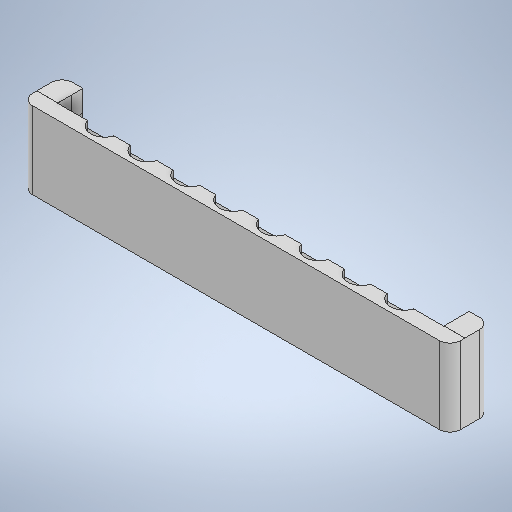
# Autodesk Inventor part: plate holder
Saved by Autodesk Inventor 2025.1 (Build 291241020, 241B)
## iProperties
Created: 2024-12-05
Part Number: plate holder
Material: Generic
Document SubType Name: Modeling
Designer: Hunter Mathis
Density: 1 g/cm^3
Appearance: Default
Author: Hunter Mathis
Autodesk Inventor part; units mm, degrees
ref_plane "YZ Plane" through (0, 0, 0) normal (1, 0, 0) x (0, 1, 0)
ref_plane "XZ Plane" through (0, 0, 0) normal (0, 1, 0) x (-1, 0, 0)
ref_plane "XY Plane" through (0, 0, 0) normal (0, 0, 1) x (1, 0, 0)
sketch "Sketch1" plane through (0, 0, 0) normal (0, 1, 0) x (-1, 0, 0)
  line L0 (63.5, -2.2225) -> (-63.5, -2.2225)
  line L1 (-63.5, -2.2225) -> (-63.5, 2.2225)
  line L2 (-63.5, 2.2225) -> (63.5, 2.2225)
  line L3 (63.5, 2.2225) -> (63.5, -2.2225)
  line L4 (63.5, -2.2225) -> (-63.5, 2.2225) construction
  line L5 (-63.5, -2.2225) -> (63.5, 2.2225) construction
  point P0 (0, 0)
  dimension "d0" = 127
  dimension "d1" = 4.445
  constraints: 12 end point, 2 midpoint, 2 parallel, 1 horizontal, 1 perpendicular
  measures "d0" distance of L1.end L2.end
  measures "d1" distance of L0.end L1.end
extrude "Extrusion1" add sketch "Sketch1" along normal blind 31.75
sketch "Sketch2" plane through (63.5, 0, -2.2225) normal (0, 0, -1) x (-1, 0, 0)
  line L0 (127, 0) -> (0, 0) projected
  line L1 (0, 0) -> (127, 0)
  line L2 (127, 0) -> (127, 25.4116)
  line L3 (127, 25.4116) -> (0, 25.4116)
  line L4 (0, 25.4116) -> (0, 0)
  point P0 (63.5, 0)
  constraints: 8 end point, 3 equal length, 1 perpendicular
extrude "Extrusion2" add sketch "Sketch2" along normal blind 7.4676
sketch "Sketch3" plane through (-63.5, 25.4116, -2.2225) normal (0, 1, 0) x (1, 0, 0)
  point P0 (63.5, -2.2225)
sketch "Sketch4" plane through (63.5, 0, -9.6901) normal (0, 0, -1) x (-1, 0, 0)
  line L0 (0, 25.4116) -> (0, 0) projected
  line L1 (6.223, 12.7058) -> (6.223, 25.4116)
  line L2 (0, 25.4116) -> (6.223, 25.4116)
  line L3 (0, 25.4116) -> (0, 12.7058)
  line L4 (0, 12.7058) -> (0, 3.1808)
  line L5 (0, 0) -> (0, 31.75) projected
  line L6 (0, 3.1808) -> (6.223, 3.1808)
  line L7 (6.223, 3.1808) -> (6.223, 12.7058)
  line L8 (0, 25.4116) -> (127, 25.4116) projected
  line L9 (127, 0) -> (127, 25.4116) projected
  line L10 (120.777, 12.7058) -> (120.777, 25.4116)
  line L11 (6.223, 25.4116) -> (120.777, 25.4116)
  line L12 (120.777, 12.7058) -> (120.777, 3.1808)
  line L13 (120.777, 3.1808) -> (127, 3.1808)
  line L14 (127, 3.1808) -> (127, 25.4116)
  line L15 (127, 0) -> (127, 31.75) projected
  line L16 (6.223, 3.1808) -> (120.777, 3.1808)
  line L17 (6.223, 3.1808) -> (6.223, 22.2308)
  line L18 (120.777, 22.2308) -> (6.223, 22.2308)
  line L19 (120.777, 22.2308) -> (120.777, 3.1808)
  line L20 (6.223, 3.1808) -> (120.777, 3.1808)
  point P0 (63.5, 0)
  point P1 (6.223, 22.2308)
  dimension "d6" = 6.223
  dimension "d7" = 9.525
  dimension "d13" = 6.223
  dimension "d14" = 19.05
  constraints: 32 end point, 5 collinear, 5 point on line, 4 perpendicular, 1 horizontal, 1 midpoint, 1 parallel, 1 vertical
  measures "d6" distance of L3.end L1.start
  measures "d7" distance of L3.end L4.end
  measures "d13" distance of L12.end L13.end
  measures "d14" distance between parallel lines of L18 L16
extrude "Extrusion3" cut sketch "Sketch4" against normal blind 4.699 contours L8 L10 L18 L1 | L18 L10 L12 L16 L7 L1
extrude "Extrusion4" add sketch "Sketch4" against normal blind 1.143 contours L18 L10 L12 L16 L7 L1
sketch "Sketch5" plane through (-63.5, 25.4116, -2.2225) normal (0, 1, 0) x (1, 0, 0)
  point P0 (63.5, -2.2225)
sketch "Sketch6" plane through (-63.5, 25.4116, -2.2225) normal (0, 1, 0) x (1, 0, 0)
  point P0 (63.5, -2.2225)
sketch "Sketch7" plane through (63.5, 0, 2.2225) normal (1, 0, 0) x (0, 0, -1)
  line L0 (0, 0) -> (0, 12.7)
  line L1 (0, 0) -> (0, 31.75) projected
  line L2 (0, 12.7) -> (11.9126, 12.7)
  line L3 (10.7696, 22.2308) -> (10.7696, 3.1808) projected
  line L4 (11.9126, 25.4116) -> (11.9126, 0) projected
  line L5 (11.9126, 12.7) -> (11.9126, 0)
  line L6 (0, 0) -> (11.9126, 0) projected
  line L7 (11.9126, 0) -> (0, 0)
  point P0 (2.2225, 0)
  dimension "d26" = 12.7
  constraints: 8 end point, 2 perpendicular, 1 collinear, 1 point on line
  measures "d26" distance of L0.start L0.end
extrude "Extrusion6" cut sketch "Sketch7" against normal through all
sketch "Sketch8" plane through (63.5, 12.7, -9.6901) normal (0, -1, 0) x (1, 0, 0)
  line L0 (-127, 11.9126) -> (0, 11.9126) projected
  line L1 (0, 7.4676) -> (0, 0) projected
  line L2 (0, 11.9126) -> (0, 0)
  line L3 (0, 0) -> (-127, 0)
  line L4 (-127, 0) -> (-127, 11.9126)
  line L5 (-127, 11.9126) -> (0, 11.9126)
  point P0 (-63.5, 9.6901)
  point P1 (-127, 11.9126)
  constraints: 8 end point, 2 parallel, 1 collinear, 1 perpendicular
extrude "Extrusion7" add sketch "Sketch8" along normal blind 3.81
sketch "Sketch9" plane through (-63.5, 25.4116, -2.2225) normal (0, 1, 0) x (1, 0, 0)
  line L0 (120.777, 2.7686) -> (6.223, 2.7686) projected
  line L1 (127, 0) -> (0, 0) projected
  line L2 (120.777, 2.7686) -> (6.5121, 2.7686)
  line L3 (6.5121, 0) -> (120.777, 0)
  line L4 (120.777, 2.7686) -> (120.777, 0)
  line L5 (120.777, 0) -> (6.223, 0)
  line L6 (6.223, 0) -> (6.223, 2.7686)
  line L7 (6.223, 2.7686) -> (120.777, 2.7686)
  line L8 (120.777, 6.3246) -> (120.777, 2.7686) projected
  point P0 (63.5, -2.2225)
  point P1 (6.223, 2.7686)
  constraints: 12 end point, 2 parallel, 1 collinear, 1 horizontal, 1 perpendicular, 1 point on line
extrude "Extrusion8" cut sketch "Sketch9" against normal blind 12.7
sketch "Sketch10" plane through (63.5, 12.7, -9.6901) normal (0, 1, 0) x (1, 0, 0)
  line L0 (-6.223, 0) -> (-6.223, -1.143) projected
  line L1 (-6.223, -1.143) -> (-6.223, -4.699) projected
  line L2 (-6.223, -1.143) -> (-6.223, -2.286)
  line L3 (-120.523, -2.286) -> (-120.523, -1.143)
  point P0 (-63.5, -9.6901)
  point P1 (-6.223, -7.4676)
  constraints: 4 end point, 1 parallel, 1 point on line
sketch "Sketch16" plane through (63.5, 0, -8.5471) normal (0, 0, 1) x (1, 0, 0)
  line L0 (-6.223, 22.2308) -> (-6.223, 12.7) projected
  line L1 (-6.223, 12.7) -> (-6.223, 22.2308)
  line L2 (-6.223, 22.2308) -> (-120.777, 22.2308)
  line L3 (-120.777, 22.2308) -> (-120.777, 12.7)
  line L4 (-120.777, 12.7) -> (-6.223, 12.7)
  point P0 (-63.5, 0)
  constraints: 8 end point, 2 parallel, 1 perpendicular, 1 vertical
extrude "Extrusion14" add sketch "Sketch16" along normal blind 2.4892
sketch "Sketch11" plane through (63.5, 8.89, -9.6901) normal (0, -1, 0) x (1, 0, 0)
  line L0 (0, 11.9126) -> (0, 7.4676) projected
  line L1 (0, 11.9126) -> (0, 7.4676)
  line L2 (0, 7.4676) -> (-6.35, 7.4676)
  line L3 (0, 11.9126) -> (-127, 11.9126) projected
  line L4 (-6.35, 11.9126) -> (-6.35, 5.5626)
  circle A0 centre (-6.35, 5.5626) radius 2.3241
  circle A1 centre (-19.05, 5.5626) radius 2.3241
  circle A2 centre (-31.75, 5.5626) radius 2.3241
  circle A3 centre (-44.45, 5.5626) radius 2.3241
  circle A4 centre (-57.15, 5.5626) radius 2.3241
  circle A5 centre (-69.85, 5.5626) radius 2.3241
  circle A6 centre (-82.55, 5.5626) radius 2.3241
  circle A7 centre (-95.25, 5.5626) radius 2.3241
  circle A8 centre (-107.95, 5.5626) radius 2.3241
  circle A9 centre (-120.65, 5.5626) radius 2.3241
  circle A10 centre (-6.35, 5.5626) radius 4.1275
  circle A11 centre (-19.05, 5.5626) radius 4.1275
  circle A12 centre (-31.75, 5.5626) radius 4.1275
  circle A13 centre (-44.45, 5.5626) radius 4.1275
  circle A14 centre (-57.15, 5.5626) radius 4.1275
  circle A15 centre (-69.85, 5.5626) radius 4.1275
  circle A16 centre (-82.55, 5.5626) radius 4.1275
  circle A17 centre (-95.25, 5.5626) radius 4.1275
  line L5 (-127, 11.9126) -> (-127, 0) projected
  line L6 (-127, 0) -> (-127, 11.9126)
  line L7 (-127, 5.9563) -> (0, 5.9563)
  circle A18 centre (-6.35, 6.35) radius 2.3241
  circle A19 centre (-19.05, 6.35) radius 2.3241
  circle A20 centre (-31.75, 6.35) radius 2.3241
  circle A21 centre (-44.45, 6.35) radius 2.3241
  circle A22 centre (-57.15, 6.35) radius 2.3241
  circle A23 centre (-69.85, 6.35) radius 2.3241
  circle A24 centre (-82.55, 6.35) radius 2.3241
  circle A25 centre (-95.25, 6.35) radius 2.3241
  circle A26 centre (-107.95, 6.35) radius 2.3241
  circle A27 centre (-120.65, 6.35) radius 2.3241
  point P0 (-63.5, 9.6901)
  dimension "d38" = 6.35
  dimension "d39" = 4.6482
  dimension "d42" = 12.7
  dimension "d51" = 8.255
  dimension "d54" = 12.7
  constraints: 28 centre point, 10 end point, 10 symmetric about line, 3 horizontal, 2 coincident, 2 perpendicular, 1 collinear, 1 midpoint, 1 point on line, 1 vertical, 42 other
  measures "d38" distance of L4.start L4.end
  measures "d39" diameter of A0
  measures "d42" distance of A0.centre A1.centre
  measures "d51" diameter of A10
  measures "d54" distance of A10.centre A11.centre
sketch "Sketch13" plane through (63.5, 12.7, -9.6901) normal (0, 1, 0) x (1, 0, 0)
  circle A0 centre (-19.05, -5.5626) radius 2.3241 projected
  circle A1 centre (-19.05, -5.5626) radius 4.1275
  line L0 (-6.223, -1.143) -> (-120.777, -1.143) projected
  line L1 (-6.223, -3.6322) -> (-6.223, -4.699) projected
  line L2 (-120.777, -4.699) -> (-120.777, -3.6322) projected
  circle A2 centre (-31.75, -5.5626) radius 4.1275
  circle A3 centre (-44.45, -5.5626) radius 4.1275
  circle A4 centre (-57.15, -5.5626) radius 4.1275
  circle A5 centre (-69.85, -5.5626) radius 4.1275
  circle A6 centre (-82.55, -5.5626) radius 4.1275
  circle A7 centre (-95.25, -5.5626) radius 4.1275
  circle A8 centre (-107.95, -5.5626) radius 4.1275
  line L3 (-6.223, -4.699) -> (-120.777, -4.699) projected
  line L4 (-6.223, -3.6322) -> (-120.777, -3.6322) projected
  line L5 (-127, -11.9126) -> (0, -11.9126) projected
  line L6 (0, 0) -> (0, -11.9126)
  line L7 (0, -11.9126) -> (0, -5.9563)
  line L8 (-127, -11.9126) -> (-127, 0) projected
  line L9 (0, -5.9563) -> (-2.9666, -5.9563)
  circle A9 centre (-19.05, -6.35) radius 2.3241
  circle A10 centre (-19.05, -6.35) radius 4.1275
  line L10 (-6.223, -10.7696) -> (-120.777, -10.7696)
  line L11 (-6.223, -8.2804) -> (-6.223, -7.2136)
  line L12 (-120.777, -7.2136) -> (-120.777, -8.2804)
  circle A11 centre (-31.75, -6.35) radius 4.1275
  circle A12 centre (-44.45, -6.35) radius 4.1275
  circle A13 centre (-57.15, -6.35) radius 4.1275
  circle A14 centre (-69.85, -6.35) radius 4.1275
  circle A15 centre (-82.55, -6.35) radius 4.1275
  circle A16 centre (-95.25, -6.35) radius 4.1275
  circle A17 centre (-107.95, -6.35) radius 4.1275
  line L13 (-6.223, -7.2136) -> (-120.777, -7.2136)
  line L14 (-6.223, -8.2804) -> (-120.777, -8.2804)
  line L15 (-127, 0) -> (-127, -11.9126)
  point P0 (-63.5, -9.6901)
  point P1 (-63.5, -2.2225)
  dimension "d59" = 8.255
  dimension "d62" = 12.7
  constraints: 18 end point, 18 symmetric about line, 17 centre point, 2 coincident, 1 horizontal, 1 midpoint, 1 vertical, 9 other
  measures "d59" diameter of A1
  measures "d62" distance of A1.centre A2.centre
fillet "Fillet1" radius 3.175 4 edges at (63.5, 20.32, 2.2225) (63.5, 17.1508, -9.6901) (-63.5, 17.1508, -9.6901) (-63.5, 20.32, 2.2225)
sketch "Sketch17" plane through (57.277, 25.4116, -2.2225) normal (0, 1, 0) x (1, 0, 0)
  line L0 (6.223, 0) -> (0, 0) projected
  line L1 (6.223, 4.2926) -> (6.223, -1.27) projected
  line L2 (6.223, 0) -> (6.223, 4.2926)
  arc A0 (6.223, 4.2926) -> (3.048, 7.4676) centre (3.048, 4.2926) ccw projected
  arc A1 (6.223, 4.2926) -> (3.048, 7.4676) centre (3.048, 4.2926) ccw
  line L3 (3.048, 7.4676) -> (0, 7.4676)
  line L4 (0, 7.4676) -> (0, 0) projected
  line L5 (0, 0) -> (6.223, 0)
  point P0 (-57.277, -2.2225)
  constraints: 6 end point, 2 point on circle, 1 centre point, 1 collinear, 1 tangent, 1 vertical
extrude "Extrusion15" add sketch "Sketch17" along normal blind 6.35
sketch "Sketch18" plane through (-63.5, 25.4116, -2.2225) normal (0, 1, 0) x (1, 0, 0)
  line L0 (127, 0) -> (0, 0) projected
  line L1 (6.2253, 0) -> (6.2253, 7.4056)
  line L2 (3.175, 7.4676) -> (6.223, 7.4676) projected
  line L3 (6.223, 7.4676) -> (3.175, 7.4676)
  arc A0 (3.175, 7.4676) -> (0, 4.2926) centre (3.175, 4.2926) ccw projected
  line L4 (0, 4.2926) -> (0, 0)
  line L5 (0, -1.27) -> (0, 4.2926) projected
  line L6 (0, 0) -> (6.2253, 0)
  arc A1 (3.175, 7.4676) -> (0, 4.2926) centre (3.175, 4.2926) ccw
  line L7 (6.223, 7.4676) -> (6.2253, 3.7028)
  line L8 (6.2253, 0) -> (0, 0)
  line L9 (0, 4.2926) -> (0, 0)
  point P0 (63.5, -2.2225)
  point P1 (15.3884, 0)
  constraints: 14 end point, 4 collinear, 3 point on circle, 1 centre point, 1 concentric, 1 horizontal, 1 midpoint, 1 point on line, 1 vertical
extrude "Extrusion16" add sketch "Sketch18" along normal blind 6.35
extrude "Extrusion17" cut sketch "Sketch11" along normal through all both and the other way through all contours L7 A1 | A19 L7 | A1 A19 | A26 A8 | A8 L7 | L7 A26 | L7 A2 | A20 L7 | A2 A20 | A25 A7 | A7 L7 | L7 A25 | L7 A3 | A21 L7 | A3 A21 | A24 A6 | A6 L7 | L7 A24 | L7 A4 | A22 L7 | A4 A22 | A23 A5 | A5 L7 | L7 A23 picked at (-19.2951, 8.1254) picked at (-108.1951, 8.1254) picked at (-31.9951, 8.1254) picked at (-95.4951, 8.1254) picked at (-44.6951, 8.1254) picked at (-82.7951, 8.1254) picked at (-57.3951, 8.1254) picked at (-70.0951, 8.1254)
ref_plane "Work Plane1" through (44.45, 22.2308, -4.1275) normal (0, 1, 0) x (1, 0, 0)
sketch "Sketch19" plane through (44.45, 22.2308, -4.1275) normal (0, 1, 0) x (1, 0, 0)
  line L0 (12.827, 1.9304) -> (-101.727, 1.9304) projected
  arc A0 (-1.6357, 0.8636) -> (-2.0377, -1.905) centre (0, -0.7874) ccw projected
  line L1 (-23.7643, 0.8636) -> (-14.3357, 0.8636) projected
  arc A1 (-1.6357, 0.8636) -> (-2.0377, -1.905) centre (0, -0.7874) ccw projected
  line L2 (-23.7643, 0.8636) -> (-14.3357, 0.8636) projected
  line L3 (-101.727, 5.5626) -> (12.827, 5.5626) projected
  line L4 (-101.727, 1.9304) -> (-101.727, 5.5626) projected
  line L5 (12.827, 5.5626) -> (12.827, 1.9304) projected
  arc A2 (-23.3623, -1.905) -> (-23.7643, 0.8636) centre (-25.4, -0.7874) ccw projected
  line L6 (-14.7377, -1.905) -> (-23.3623, -1.905) projected
  arc A3 (-14.3357, 0.8636) -> (-14.7377, -1.905) centre (-12.7, -0.7874) ccw projected
  arc A4 (-74.1623, -1.905) -> (-74.5643, 0.8636) centre (-76.2, -0.7874) ccw projected
  line L7 (-65.5377, -1.905) -> (-74.1623, -1.905) projected
  arc A5 (-65.1357, 0.8636) -> (-65.5377, -1.905) centre (-63.5, -0.7874) ccw projected
  line L8 (-74.5643, 0.8636) -> (-65.1357, 0.8636) projected
  arc A6 (-61.4623, -1.905) -> (-61.8643, 0.8636) centre (-63.5, -0.7874) ccw projected
  line L9 (-52.8377, -1.905) -> (-61.4623, -1.905) projected
  arc A7 (-52.4357, 0.8636) -> (-52.8377, -1.905) centre (-50.8, -0.7874) ccw projected
  line L10 (-61.8643, 0.8636) -> (-52.4357, 0.8636) projected
  arc A8 (-10.6623, -1.905) -> (-11.0643, 0.8636) centre (-12.7, -0.7874) ccw projected
  line L11 (-2.0377, -1.905) -> (-10.6623, -1.905) projected
  line L12 (-11.0643, 0.8636) -> (-1.6357, 0.8636) projected
  arc A9 (-27.0357, 0.8636) -> (-27.4377, -1.905) centre (-25.4, -0.7874) ccw projected
  line L13 (-36.4643, 0.8636) -> (-27.0357, 0.8636) projected
  arc A10 (-36.0623, -1.905) -> (-36.4643, 0.8636) centre (-38.1, -0.7874) ccw projected
  line L14 (-27.4377, -1.905) -> (-36.0623, -1.905) projected
  arc A11 (-77.8357, 0.8636) -> (-78.2377, -1.905) centre (-76.2, -0.7874) ccw projected
  line L15 (-87.2643, 0.8636) -> (-77.8357, 0.8636) projected
  arc A12 (-86.8623, -1.905) -> (-87.2643, 0.8636) centre (-88.9, -0.7874) ccw projected
  line L16 (-78.2377, -1.905) -> (-86.8623, -1.905) projected
  arc A13 (-39.7357, 0.8636) -> (-40.1377, -1.905) centre (-38.1, -0.7874) ccw projected
  line L17 (-49.1643, 0.8636) -> (-39.7357, 0.8636) projected
  arc A14 (-48.7623, -1.905) -> (-49.1643, 0.8636) centre (-50.8, -0.7874) ccw projected
  line L18 (-40.1377, -1.905) -> (-48.7623, -1.905) projected
  arc A15 (2.0377, -1.905) -> (1.6357, 0.8636) centre (0, -0.7874) ccw projected
  line L19 (12.827, -1.905) -> (2.0377, -1.905) projected
  line L20 (12.827, 0.8636) -> (12.827, -1.905) projected
  line L21 (1.6357, 0.8636) -> (12.827, 0.8636) projected
  arc A16 (-90.5357, 0.8636) -> (-90.9377, -1.905) centre (-88.9, -0.7874) ccw projected
  line L22 (-101.727, 0.8636) -> (-90.5357, 0.8636) projected
  line L23 (-101.727, -1.905) -> (-101.727, 0.8636) projected
  line L24 (-90.9377, -1.905) -> (-101.727, -1.905) projected
  arc A17 (-23.3623, -1.905) -> (-23.7643, 0.8636) centre (-25.4, -0.7874) ccw projected
  line L25 (-14.7377, -1.905) -> (-23.3623, -1.905) projected
  arc A18 (-14.3357, 0.8636) -> (-14.7377, -1.905) centre (-12.7, -0.7874) ccw projected
  arc A19 (-74.1623, -1.905) -> (-74.5643, 0.8636) centre (-76.2, -0.7874) ccw projected
  line L26 (-65.5377, -1.905) -> (-74.1623, -1.905) projected
  arc A20 (-65.1357, 0.8636) -> (-65.5377, -1.905) centre (-63.5, -0.7874) ccw projected
  line L27 (-74.5643, 0.8636) -> (-65.1357, 0.8636) projected
  arc A21 (-61.4623, -1.905) -> (-61.8643, 0.8636) centre (-63.5, -0.7874) ccw projected
  line L28 (-52.8377, -1.905) -> (-61.4623, -1.905) projected
  arc A22 (-52.4357, 0.8636) -> (-52.8377, -1.905) centre (-50.8, -0.7874) ccw projected
  line L29 (-61.8643, 0.8636) -> (-52.4357, 0.8636) projected
  arc A23 (-10.6623, -1.905) -> (-11.0643, 0.8636) centre (-12.7, -0.7874) ccw projected
  line L30 (-2.0377, -1.905) -> (-10.6623, -1.905) projected
  line L31 (-11.0643, 0.8636) -> (-1.6357, 0.8636) projected
  arc A24 (-27.0357, 0.8636) -> (-27.4377, -1.905) centre (-25.4, -0.7874) ccw projected
  line L32 (-36.4643, 0.8636) -> (-27.0357, 0.8636) projected
  arc A25 (-36.0623, -1.905) -> (-36.4643, 0.8636) centre (-38.1, -0.7874) ccw projected
  line L33 (-27.4377, -1.905) -> (-36.0623, -1.905) projected
  arc A26 (-77.8357, 0.8636) -> (-78.2377, -1.905) centre (-76.2, -0.7874) ccw projected
  line L34 (-87.2643, 0.8636) -> (-77.8357, 0.8636) projected
  arc A27 (-86.8623, -1.905) -> (-87.2643, 0.8636) centre (-88.9, -0.7874) ccw projected
  line L35 (-78.2377, -1.905) -> (-86.8623, -1.905) projected
  arc A28 (-39.7357, 0.8636) -> (-40.1377, -1.905) centre (-38.1, -0.7874) ccw projected
  line L36 (-49.1643, 0.8636) -> (-39.7357, 0.8636) projected
  arc A29 (-48.7623, -1.905) -> (-49.1643, 0.8636) centre (-50.8, -0.7874) ccw projected
  line L37 (-40.1377, -1.905) -> (-48.7623, -1.905) projected
  arc A30 (2.0377, -1.905) -> (1.6357, 0.8636) centre (0, -0.7874) ccw projected
  line L38 (12.827, -1.905) -> (2.0377, -1.905) projected
  line L39 (12.827, 0.8636) -> (12.827, -1.905) projected
  line L40 (1.6357, 0.8636) -> (12.827, 0.8636) projected
  arc A31 (-90.5357, 0.8636) -> (-90.9377, -1.905) centre (-88.9, -0.7874) ccw projected
  line L41 (-101.727, 0.8636) -> (-90.5357, 0.8636) projected
  line L42 (-101.727, -1.905) -> (-101.727, 0.8636) projected
  line L43 (-90.9377, -1.905) -> (-101.727, -1.905) projected
  point P0 (-44.45, -4.1275)
extrude "Extrusion19" cut sketch "Sketch13" along normal blind 19.05 and the other way blind 2.54 contours A0 A9 L3 | A0 L3 A10 A1 L13 A9 | L3 A9 A0 L4 | A0 L4 A10 L3 | A9 L13 A0 | A0 L13 A9 L3 | L4 A0 | A0 L4 A10 | L3 A9 | L13 A9 L14 A0 | A0 L13 | A0 L3 A10 L4 | A10 L13 A1 | A9 A0 L3 | L13 A9 A0 | L13 A1 L14 A9 | A0 A9 L13 A1 A10 L3 | L13 A10 L14 A1 | A9 L14 A1 L13 | L14 A1 A9 | A9 L14 | L14 A10 A1 | L13 A10 A1 | A1 L14 A10 L13 | A11 L3 L4 | L4 A11 | L13 A2 A11 | A11 L14 A2 L13 | A11 A2 L13 L3 | A11 L14 A2 | A2 L14 L13 | A2 L13 A11 | A12 L3 L4 | L4 A12 | A11 L13 A2 L14 | A2 L14 | A12 A3 L13 L3 | L14 A3 L13 A12 | A12 L14 A3 | L13 A3 A12 | A3 L13 A12 | A13 L3 L4 | L4 A13 | A12 L13 A3 L14 | L14 A3 L13 | A3 L14 | A13 A4 L13 L3 | L14 A4 L13 A13 | A13 L14 A4 | L13 A4 A13 | A4 L13 A13 | A14 L3 L4 | L4 A14 | A13 L13 A4 L14 | L14 A4 L13 | A4 L14 | A14 A5 L13 L3 | L14 A5 L13 A14 | A14 L14 A5 | L13 A5 A14 | A5 L13 A14 | A15 L3 L4 | L4 A15 | A14 L13 A5 L14 | L14 A5 L13 | A5 L14 | A15 A6 L13 L3 | L14 A6 L13 A15 | A15 L14 A6 | L13 A6 A15 | A6 L13 A15 | A16 L3 L4 | L4 A16 | A15 L13 A6 L14 | L14 A6 L13 | A6 L14 | A16 A7 L13 L3 | L14 A7 L13 A16 | A16 L14 A7 | L13 A7 A16 | A7 L13 A16 | A17 L3 L4 | L4 A17 | A16 L13 A7 L14 | L14 A7 L13 | A7 L14 | A17 A8 L13 L3 | L14 A8 L13 A17 | A17 L14 A8 | L13 A8 A17 | A8 L13 A17 | A17 L13 A8 L14 | L14 A8 L13 | A8 L14
sketch "Sketch20" plane through (63.5, 12.7, -9.6901) normal (0, 1, 0) x (1, 0, 0)
  arc A0 (-60.2564, -3.6322) -> (-60.9329, -4.699) centre (-57.15, -6.35) ccw projected
  line L0 (-60.2564, -3.6322) -> (-66.7436, -3.6322) projected
  arc A1 (-66.0671, -4.699) -> (-66.7436, -3.6322) centre (-69.85, -6.35) ccw projected
  line L1 (-60.9329, -4.699) -> (-66.0671, -4.699) projected
  arc A2 (-47.5564, -3.6322) -> (-48.2329, -4.699) centre (-44.45, -6.35) ccw projected
  line L2 (-47.5564, -3.6322) -> (-54.0436, -3.6322) projected
  arc A3 (-53.3671, -4.699) -> (-54.0436, -3.6322) centre (-57.15, -6.35) ccw projected
  line L3 (-48.2329, -4.699) -> (-53.3671, -4.699) projected
  arc A4 (-40.6671, -4.699) -> (-41.3436, -3.6322) centre (-44.45, -6.35) ccw projected
  line L4 (-35.5329, -4.699) -> (-40.6671, -4.699) projected
  arc A5 (-34.8564, -3.6322) -> (-35.5329, -4.699) centre (-31.75, -6.35) ccw projected
  line L5 (-34.8564, -3.6322) -> (-41.3436, -3.6322) projected
  arc A6 (-27.9671, -4.699) -> (-28.6436, -3.6322) centre (-31.75, -6.35) ccw projected
  line L6 (-22.8329, -4.699) -> (-27.9671, -4.699) projected
  arc A7 (-22.1564, -3.6322) -> (-22.8329, -4.699) centre (-19.05, -6.35) ccw projected
  line L7 (-22.1564, -3.6322) -> (-28.6436, -3.6322) projected
  arc A8 (-15.2671, -4.699) -> (-15.9436, -3.6322) centre (-19.05, -6.35) ccw projected
  line L8 (-6.223, -4.699) -> (-15.2671, -4.699) projected
  line L9 (-6.223, -3.6322) -> (-6.223, -4.699) projected
  line L10 (-6.223, -3.6322) -> (-15.9436, -3.6322) projected
  arc A9 (-78.7671, -4.699) -> (-79.4436, -3.6322) centre (-82.55, -6.35) ccw projected
  line L11 (-73.6329, -4.699) -> (-78.7671, -4.699) projected
  arc A10 (-72.9564, -3.6322) -> (-73.6329, -4.699) centre (-69.85, -6.35) ccw projected
  line L12 (-72.9564, -3.6322) -> (-79.4436, -3.6322) projected
  arc A11 (-91.4671, -4.699) -> (-92.1436, -3.6322) centre (-95.25, -6.35) ccw projected
  line L13 (-86.3329, -4.699) -> (-91.4671, -4.699) projected
  arc A12 (-85.6564, -3.6322) -> (-86.3329, -4.699) centre (-82.55, -6.35) ccw projected
  line L14 (-85.6564, -3.6322) -> (-92.1436, -3.6322) projected
  arc A13 (-98.3564, -3.6322) -> (-99.0329, -4.699) centre (-95.25, -6.35) ccw projected
  line L15 (-98.3564, -3.6322) -> (-104.8436, -3.6322) projected
  arc A14 (-104.1671, -4.699) -> (-104.8436, -3.6322) centre (-107.95, -6.35) ccw projected
  line L16 (-99.0329, -4.699) -> (-104.1671, -4.699) projected
  arc A15 (-111.0564, -3.6322) -> (-111.7329, -4.699) centre (-107.95, -6.35) ccw projected
  line L17 (-111.0564, -3.6322) -> (-120.777, -3.6322) projected
  line L18 (-120.777, -4.699) -> (-120.777, -3.6322) projected
  line L19 (-111.7329, -4.699) -> (-120.777, -4.699) projected
  point P0 (-63.5, -9.6901)
extrude "Extrusion20" add sketch "Sketch20" along normal up to surface (0.0116 mm away)
sketch "Sketch21" plane through (0, 31.75, 0) normal (0, 1, 0) x (1, 0, 0)
  arc A0 (15.0767, 2.2225) -> (23.0233, 2.2225) centre (19.05, 3.3401) ccw projected
  line L0 (15.0767, 2.2225) -> (10.3233, 2.2225) projected
  arc A1 (2.3767, 2.2225) -> (10.3233, 2.2225) centre (6.35, 3.3401) ccw projected
  line L1 (2.3767, 2.2225) -> (-2.3767, 2.2225) projected
  arc A2 (-10.3233, 2.2225) -> (-2.3767, 2.2225) centre (-6.35, 3.3401) ccw projected
  line L2 (-10.3233, 2.2225) -> (-15.0767, 2.2225) projected
  arc A3 (-23.0233, 2.2225) -> (-15.0767, 2.2225) centre (-19.05, 3.3401) ccw projected
  line L3 (-23.0233, 2.2225) -> (-27.7767, 2.2225) projected
  arc A4 (-35.7233, 2.2225) -> (-27.7767, 2.2225) centre (-31.75, 3.3401) ccw projected
  line L4 (-35.7233, 2.2225) -> (-40.4767, 2.2225) projected
  arc A5 (-48.4233, 2.2225) -> (-40.4767, 2.2225) centre (-44.45, 3.3401) ccw projected
  line L5 (-48.4233, 2.2225) -> (-57.2747, 2.2225) projected
  line L6 (-57.2747, 2.2225) -> (-63.5, 2.2225) projected
  line L7 (-63.5, 2.2225) -> (-63.5, 0.9525) projected
  arc A6 (-63.5, 0.9525) -> (-60.325, -2.2225) centre (-60.325, 0.9525) ccw projected
  line L8 (-60.325, -2.2225) -> (60.325, -2.2225) projected
  arc A7 (60.325, -2.2225) -> (63.5, 0.9525) centre (60.325, 0.9525) ccw projected
  line L9 (63.5, 0.9525) -> (63.5, 2.2225) projected
  line L10 (63.5, 2.2225) -> (57.277, 2.2225) projected
  line L11 (57.277, 2.2225) -> (48.4233, 2.2225) projected
  arc A8 (40.4767, 2.2225) -> (48.4233, 2.2225) centre (44.45, 3.3401) ccw projected
  line L12 (40.4767, 2.2225) -> (35.7233, 2.2225) projected
  arc A9 (27.7767, 2.2225) -> (35.7233, 2.2225) centre (31.75, 3.3401) ccw projected
  line L13 (27.7767, 2.2225) -> (23.0233, 2.2225) projected
  arc A10 (22.1564, 6.0579) -> (15.9436, 6.0579) centre (19.05, 3.3401) ccw projected
  line L14 (28.6436, 6.0579) -> (22.1564, 6.0579) projected
  arc A11 (34.8564, 6.0579) -> (28.6436, 6.0579) centre (31.75, 3.3401) ccw projected
  line L15 (41.3436, 6.0579) -> (34.8564, 6.0579) projected
  arc A12 (47.5564, 6.0579) -> (41.3436, 6.0579) centre (44.45, 3.3401) ccw projected
  line L16 (57.277, 6.0579) -> (47.5564, 6.0579) projected
  line L17 (57.277, 9.6901) -> (57.277, 6.0579) projected
  line L18 (-57.277, 9.6901) -> (57.277, 9.6901) projected
  line L19 (-57.277, 6.0579) -> (-57.277, 9.6901) projected
  line L20 (-47.5564, 6.0579) -> (-57.277, 6.0579) projected
  arc A13 (-41.3436, 6.0579) -> (-47.5564, 6.0579) centre (-44.45, 3.3401) ccw projected
  line L21 (-34.8564, 6.0579) -> (-41.3436, 6.0579) projected
  arc A14 (-28.6436, 6.0579) -> (-34.8564, 6.0579) centre (-31.75, 3.3401) ccw projected
  line L22 (-22.1564, 6.0579) -> (-28.6436, 6.0579) projected
  arc A15 (-15.9436, 6.0579) -> (-22.1564, 6.0579) centre (-19.05, 3.3401) ccw projected
  line L23 (-9.4564, 6.0579) -> (-15.9436, 6.0579) projected
  arc A16 (-3.2436, 6.0579) -> (-9.4564, 6.0579) centre (-6.35, 3.3401) ccw projected
  line L24 (3.2436, 6.0579) -> (-3.2436, 6.0579) projected
  arc A17 (9.4564, 6.0579) -> (3.2436, 6.0579) centre (6.35, 3.3401) ccw projected
  line L25 (15.9436, 6.0579) -> (9.4564, 6.0579) projected
  line L26 (57.277, 2.2225) -> (63.5, 2.2225) projected
  line L27 (63.5, 2.2225) -> (63.5, 6.5151) projected
  arc A18 (63.5, 6.5151) -> (60.325, 9.6901) centre (60.325, 6.5151) ccw projected
  line L28 (60.325, 9.6901) -> (57.277, 9.6901) projected
  line L29 (57.277, 9.6901) -> (57.277, 2.2225) projected
  line L30 (-57.277, 9.6901) -> (-60.325, 9.6901) projected
  arc A19 (-60.325, 9.6901) -> (-63.5, 6.5151) centre (-60.325, 6.5151) ccw projected
  line L31 (-63.5, 6.5151) -> (-63.5, 2.2225) projected
  line L32 (-63.5, 2.2225) -> (-57.2747, 2.2225) projected
  line L33 (-57.2747, 2.2225) -> (-57.2747, 5.9253) projected
  line L34 (-57.2747, 5.9253) -> (-57.277, 9.6901) projected
  line L35 (57.277, 2.2225) -> (57.277, 6.0579)
  line L36 (57.277, 2.2225) -> (57.277, 4.1402)
  line L37 (57.277, 4.1402) -> (57.277, 6.1722)
  line L38 (57.277, 9.6901) -> (57.277, 2.2225) projected
  line L39 (57.277, 6.1722) -> (57.277, 2.1082)
  line L40 (57.277, 2.1082) -> (-57.2749, 2.1082)
  line L41 (-57.2749, 2.1082) -> (-57.2749, 6.1722)
  line L42 (-57.2749, 6.1722) -> (57.277, 6.1722)
  line L43 (57.277, 6.1722) -> (57.277, 2.1082)
  point P0 (0, 0)
  dimension "d90" = 2.032
  dimension "d91" = 4.064
  constraints: 16 end point, 3 point on line, 2 parallel, 1 collinear, 1 horizontal, 1 midpoint, 1 perpendicular
  measures "d90" distance of L36.end L37.end
  measures "d91" distance of L37.end L39.end
extrude "Extrusion21" cut sketch "Sketch21" against normal up to surface (19.0384 mm away) contours L0 A1 L40 L1 A2 L2 A3 L3 A4 L4 A5 L5 L33 L34 L20 A13 L42 L21 A14 L22 A15 L23 A16 L24 A17 L25 A10 L14 A11 L15 A12 L16 L29 L11 A8 L12 A9 L13 A0 | A0 L40 A1 L0 | A0 L13 A9 L40 | L40 A2 L1 A1 | A9 L12 A8 L40 | L40 A3 L2 A2 | A8 L11 L39 L40 | L40 A4 L3 A3 | L40 A5 L4 A4 | L16 A12 L42 L17 | L40 L41 L5 A5 | A12 L15 A11 L42 | L42 A13 L20 L19 | A11 L14 A10 L42 | L42 A14 L21 A13 | A10 L25 A17 L42 | L42 A15 L22 A14 | A17 L24 A16 L42 | L42 A16 L23 A15
body "Solid1"
